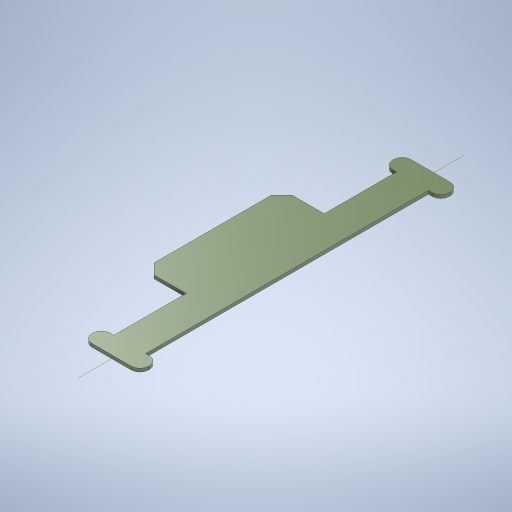
# Autodesk Inventor part: linefollower_chassy_model
Saved by Autodesk Inventor 2024 (Build 280153000, 153)
## iProperties
Created: 2024-02-06
Part Number: linefollower_chassy_model
Material: Generic
Document SubType Name: Modeling
Designer: kamil
Density: 1 g/cm^3
Appearance: Default
Author: kamil
Autodesk Inventor part; units mm, degrees
ref_plane "YZ Plane" through (0, 0, 0) normal (1, 0, 0) x (0, 1, 0)
ref_plane "XZ Plane" through (0, 0, 0) normal (0, 1, 0) x (-1, 0, 0)
ref_plane "XY Plane" through (0, 0, 0) normal (0, 0, 1) x (1, 0, 0)
sketch "Sketch1" plane through (0, 0, 0) normal (0, 1, 0) x (-1, 0, 0)
  line L0 (7.5, 75) -> (-7.5, 75)
  line L1 (-7.5, 75) -> (-7.5, -75)
  line L2 (-7.5, -75) -> (7.5, -75)
  line L3 (7.5, -75) -> (7.5, 75)
  line L4 (-7.5, 75) -> (7.5, -75) construction
  line L5 (-7.5, -75) -> (7.5, 75) construction
  line L6 (7.5, -66.5) -> (9.3, -66.5)
  line L7 (13.3, -70.5) -> (13.3, -71)
  line L8 (9.3, -75) -> (7.5, -75)
  line L9 (7.5, -75) -> (7.5, -66.5)
  arc A0 (13.3, -70.5) -> (9.3, -66.5) centre (9.3, -70.5) ccw
  arc A1 (9.3, -75) -> (13.3, -71) centre (9.3, -71) ccw
  line L10 (0, 75) -> (0, -75) construction
  line L11 (-7.5, -66.5) -> (-9.3, -66.5)
  line L12 (-13.3, -70.5) -> (-13.3, -71)
  line L13 (-9.3, -75) -> (-7.5, -75)
  arc A2 (-9.3, -66.5) -> (-13.3, -70.5) centre (-9.3, -70.5) ccw
  arc A3 (-13.3, -71) -> (-9.3, -75) centre (-9.3, -71) ccw
  line L14 (-7.5, 0) -> (7.5, 0) construction
  line L15 (7.5, 66.5) -> (9.3, 66.5)
  line L16 (13.3, 70.5) -> (13.3, 71)
  line L17 (9.3, 75) -> (7.5, 75)
  arc A4 (9.3, 66.5) -> (13.3, 70.5) centre (9.3, 70.5) ccw
  arc A5 (13.3, 71) -> (9.3, 75) centre (9.3, 71) ccw
  arc A6 (-13.3, 70.5) -> (-9.3, 66.5) centre (-9.3, 70.5) ccw
  line L18 (-13.3, 70.5) -> (-13.3, 71)
  arc A7 (-9.3, 75) -> (-13.3, 71) centre (-9.3, 71) ccw
  line L19 (-9.3, 75) -> (-7.5, 75)
  line L20 (-7.5, 66.5) -> (-9.3, 66.5)
  line L21 (7.5, -20.0447) -> (7.5, 20.0447)
  line L22 (7.5, 32.5) -> (22.5, 32.5)
  line L23 (27.5, 27.5) -> (27.5, -27.5)
  line L24 (22.5, -32.5) -> (7.5, -32.5)
  line L25 (7.5, -32.5) -> (7.5, 32.5)
  line L26 (-7.5, 1.5) -> (-14.5, 1.5)
  line L27 (-14.5, 1.5) -> (-14.5, -1.5)
  line L28 (-14.5, -1.5) -> (-7.5, -1.5)
  line L29 (-7.5, -1.5) -> (-7.5, 1.5)
  circle A8 centre (-12.5, 0) radius 0.98
  line L30 (22.5, -32.5) -> (27.5, -27.5)
  line L31 (22.5, 32.5) -> (27.5, 27.5)
  point P0 (0, 0)
  point P1 (0, 0)
  point P2 (13.3, -75)
  point P3 (13.3, -66.5)
  point P4 (0, 0)
  point P5 (27.5, -32.5)
  point P6 (27.5, 32.5)
  point P7 (27.5, 0)
  point P8 (0, 0)
  point P9 (-11, -1.5)
  point P10 (-14.5, 0)
  point P11 (-7.5, 0)
  point P12 (7.5, -32.5)
  dimension "d0" = 150
  dimension "d1" = 15
  dimension "d2" = 5.8
  dimension "d3" = 8.5
  dimension "d4" = 4
  dimension "d5" = 20
  dimension "d6" = 65
  dimension "d7" = 1.96
  dimension "d8" = 3
  dimension "d9" = 7
  dimension "d10" = 5
  dimension "d11" = 5
  dimension "d12" = 5
  dimension "d13" = 5
  dimension "d14" = 5
  dimension "d17" = 1.8
  dimension "d18" = 0.5
  dimension "d19" = 4
  dimension "d20" = 4
  constraints: 64 end point, 21 symmetric about line, 16 point on circle, 12 point on line, 11 midpoint, 9 centre point, 8 parallel, 4 horizontal, 4 perpendicular, 4 tangent, 3 horizontal alignment, 1 coincident, 1 equal radius, 6 other
  measures "d0" distance of L2.end L0.start
  measures "d1" distance between parallel lines of L1 L3
  measures "d2" distance of L2.end point (13.3, -75)
  measures "d3" distance of point (13.3, -66.5) point (13.3, -75)
  measures "d4" radius of A0
  measures "d5" distance of point (27.5, -32.5) L24.end
  measures "d6" distance of point (27.5, 32.5) point (27.5, -32.5)
  measures "d7" diameter of A8
  measures "d8" distance from line of point (-11, -1.5) L26
  measures "d9" distance between parallel lines of L1 L27
  measures "d10" distance of point (-7.5, 0) A8.centre
  measures "d11" distance of L24.start point (27.5, -32.5)
  measures "d12" distance of L23.end point (27.5, -32.5)
  measures "d13" distance of L22.end point (27.5, 32.5)
  measures "d14" distance of L23.start point (27.5, 32.5)
  measures "d17" distance of L8.start L2.end
  measures "d18" distance of L7.start L7.end
  measures "d19" radius of A1
  measures "d20" distance from line of L8 A1.centre
extrude "Extrusion1" add sketch "Sketch1" along normal blind 1.57 contours L3 L2 L1 L0 | L17 A5 L16 A4 L15 L3 | L1 L20 A6 L18 A7 L19 | L22 L31 L23 L30 L24 L3 | L1 L13 A3 L12 A2 L11 | L6 A0 L7 A1 L8 L3
equation "\"d12\" = d11"
equation "\"d13\" = d11"
equation "\"d14\" = d13"
body "Solid1"
